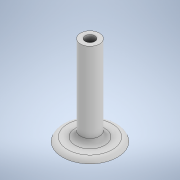
# Autodesk Inventor part: flume-nursery
Saved by Autodesk Inventor 2021 (Build 250183000, 183)
## iProperties
Created: 2020-08-01
Part Number: flume-nursery
Material: Generic
Document SubType Name: Modeling
Designer: Scratch
Density: 1 g/cm^3
Appearance: Default
Author: Scratch
Autodesk Inventor part; units mm, degrees
ref_plane "YZ Plane" through (0, 0, 0) normal (1, 0, 0) x (0, 1, 0)
ref_plane "XZ Plane" through (0, 0, 0) normal (0, 1, 0) x (-1, 0, 0)
ref_plane "XY Plane" through (0, 0, 0) normal (0, 0, 1) x (1, 0, 0)
sketch "Sketch1" plane through (0, 0, 0) normal (0, 0, 1) x (1, 0, 0)
  line L0 (1.1948, 21.5189) -> (2.2959, 21.5189)
  line L1 (6.6309, 0) -> (1.1948, 0)
  line L2 (1.1948, 0.9728) -> (1.1948, 21.5189)
  line L3 (2.2959, 21.5189) -> (2.2959, 0.9728)
  line L4 (2.2959, 0.9728) -> (6.6309, 0.9728)
  line L5 (6.6309, 0.9728) -> (6.6309, 0)
  line L6 (1.1948, 0.9728) -> (0, 0.9728)
  line L7 (0, 0.9728) -> (0, 0)
  line L8 (0, 0) -> (1.1948, 0)
  constraints: 18 end point, 2 horizontal, 2 perpendicular, 2 point on line, 1 parallel, 1 vertical
revolve "Revolution1" add sketch "Sketch1" angle 360 about axis through (0, 0.9728, 0) along (0, -1, 0)
fillet "Fillet1" radius 1.27 1 edges at (-2.2959, 0.9728, 0)
fillet "Fillet2" radius 1.27 1 edges at (-6.6309, 0.9728, 0)
body "Solid1"
